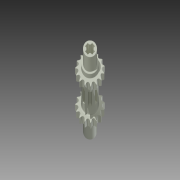
# Autodesk Inventor part: 1
Saved by Autodesk Inventor 2015 (Build 190159000, 159)
## iProperties
Created: 2016-01-25
Part Number: 1
Material: Plástico ABS
Document SubType Name: Modeling
Designer: Javier Pérez de Frutos
Density: 1.06 g/cm^3
Appearance: Suave - Marfil
z: 15,000 su
deje: 1,600 mm
rcanal: 0,500 mm
Dint: 13,500 mm
r3: 12,475 mm
Dcanal: 10,000 mm
Lcanal: 10,000 mm
L: 15,000 mm
Dext: 16,842 mm
Dr: 1,500 mm
Dp: 15,000 mm
r1: 1,124 mm
r2: 3,960 mm
chi: 124,00 gr
tau: 24,00 gr
p: 3,119 mm
Author: Javier Pérez de Frutos
Title: Piñón Tractor
Autodesk Inventor part; units mm, degrees
ref_plane "YZ Plane" through (0, 0, 0) normal (1, 0, 0) x (0, 1, 0)
ref_plane "XZ Plane" through (0, 0, 0) normal (0, 1, 0) x (-1, 0, 0)
ref_plane "XY Plane" through (0, 0, 0) normal (0, 0, 1) x (1, 0, 0)
sketch "Base" plane through (0, 0, 0) normal (0, 0, 1) x (1, 0, 0)
  circle A0 centre (0, 0) radius 7.5
  dimension "d0" = 15
  constraints: 1 centre point, 1 coincident
  measures "d0" diameter of A0
sketch "Tooth_drawing" plane through (0, 0, 0) normal (0, 0, 1) x (1, 0, 0)
  line L0 (0, 9) -> (0, -9)
  line L1 (-9, 0) -> (9, 0)
  line L2 (0, 0) -> (-1.7508, 8.2371)
  line L3 (0, 0) -> (1.7508, 8.2371)
  circle A0 centre (0, 7.5) radius 0.75
  arc A1 (-0.9925, 7.3464) -> (0.9925, 7.3464) centre (0, 7.8741) ccw
  line L4 (0, 7.8741) -> (-0.9925, 7.3464)
  line L5 (0, 7.8741) -> (0.9925, 7.3464)
  circle A2 centre (0, 0) radius 8.4211
  arc A3 (-0.9925, 7.3464) -> (-1.6459, 8.2587) centre (-4.7327, 5.3577) ccw
  arc A4 (1.6459, 8.2587) -> (0.9925, 7.3464) centre (4.7327, 5.3577) ccw
  dimension "d17" = 12
  dimension "d18" = 12
  dimension "d19" = 7.5
  dimension "d20" = 1.5
  dimension "d21" = 2.2482
  dimension "d22" = 62
  dimension "d23" = 62
  dimension "d25" = 16.8422
  constraints: 12 end point, 10 point on circle, 5 centre point, 3 point on line, 2 coincident, 2 midpoint, 2 tangent, 1 perpendicular, 1 vertical
  measures "d17" angle of L2 L0
  measures "d18" angle of L0 L3
  measures "d19" distance of point (0, 0) A0.centre
  measures "d20" diameter of A0
  measures "d21" diameter of A1
  measures "d22" angle of L0 L4
  measures "d23" angle of L0 L5
  measures "d25" diameter of A2
extrude "Tooth" add sketch "Tooth_drawing" along normal mid plane 15 contours A2 L3 L0 A1 A4 | A3 A1 L0 L2 A2
pattern_circular "Teeth" count 15 over 360 about axis through (0, 0, -10) along (0, 0, 1) of "Tooth"
sketch "Canal_drawing" plane through (0, 0, 0) normal (0, 1, 0) x (-1, 0, 0)
  line L0 (7.7013, 0) -> (-7.7013, 0)
  line L1 (-5.5, 5) -> (-6.75, 5)
  line L2 (-5, 4.5) -> (-5, 0)
  arc A0 (-8.4211, 5.228) -> (-6.75, 5) centre (-6.75, 11.2374) ccw
  line L3 (0, 7.5) -> (-6.75, 7.5)
  line L4 (0, 0) -> (0, 7.5)
  arc A1 (-6.75, 7.5) -> (-8.4211, 7.1913) centre (-6.75, 2.822) ccw
  line L5 (1.3412, 6.25) -> (-12.5756, 6.25)
  line L6 (-8.4211, 7.1913) -> (-8.4211, 5.228)
  line L7 (-5.5, -5) -> (-6.75, -5)
  line L8 (-5, -4.5) -> (-5, 0)
  arc A2 (-6.75, -5) -> (-8.4211, -5.228) centre (-6.75, -11.2374) ccw
  line L9 (0, -7.5) -> (-6.75, -7.5)
  line L10 (0, 0) -> (0, -7.5)
  arc A3 (-8.4211, -7.1913) -> (-6.75, -7.5) centre (-6.75, -2.822) ccw
  line L11 (-8.4211, -7.1913) -> (-8.4211, -5.228)
  line L12 (0, -15.7323) -> (0, 15.7323) projected
  arc A4 (-5.5, -5) -> (-5, -4.5) centre (-5.5, -4.5) ccw
  arc A5 (-5, 4.5) -> (-5.5, 5) centre (-5.5, 4.5) ccw
  point P0 (0, 0)
  point P1 (-5, 5)
  point P2 (-5, -5)
  dimension "d48" = 5
  dimension "d50" = 12.4747
  dimension "d53" = 6.75
  dimension "d54" = 6.75
  dimension "d56" = 6.75
  dimension "d57" = 4.678
  dimension "d58" = 12.5
  dimension "d59" = 8.4211
  dimension "d60" = 5
  dimension "d61" = 15
  dimension "d63" = 0.5
  constraints: 24 end point, 12 point on circle, 8 symmetric about line, 6 centre point, 6 tangent, 5 point on line, 4 horizontal, 2 midpoint, 1 coincident, 1 equal radius, 1 perpendicular, 1 vertical, 2 other
  measures "d48" distance from line of point (0, 0) L2
  measures "d50" diameter of A0
  measures "d53" distance from line of L4 A0.centre
  measures "d54" distance from line of L1.end L4
  measures "d56" horizontal distance of point (0, 0) A1.centre
  measures "d57" radius of A1
  measures "d58" diameter of L5.start L0
  measures "d59" distance from line of L6.start L4
  measures "d60" distance of point (-5, 5) L2.end
  measures "d61" diameter of L3 L0
  measures "d63" radius of A4
revolve "Canal" cut sketch "Canal_drawing" angle 360 about axis through (0, 0, -10) along (0, 0, 1) keep common part
sketch "Axis_drawing" plane through (0, 0, 0) normal (0, 0, 1) x (1, 0, 0)
  arc A0 (-1.6, -1.2) -> (-1.6, 1.2) centre (0, 0) ccw
  line L0 (-1.6, 1.2) -> (-1.6, -1.2)
  dimension "d64" = 4
  dimension "d65" = 1.6
  constraints: 2 end point, 2 point on circle, 1 centre point, 1 coincident, 1 vertical
  measures "d64" diameter of A0
  measures "d65" distance from line of point (0, 0) L0
extrude "Axis" [suppressed]
sketch "Holes_drawing" plane through (0, 0, 0) normal (0, 0, 1) x (1, 0, 0)
  circle A0 centre (0, 0) radius 5 projected
  circle A1 centre (0, 0) radius 5 projected
  arc A2 (-1.6, -1.2) -> (-1.6, 1.2) centre (0, 0) ccw projected
  line L0 (1.9182, -4.6174) -> (0.7673, -1.847)
  circle A3 centre (0, 0) radius 3.5
  circle A4 centre (-3.5, 0) radius 0.75
  circle A5 centre (-1.75, -3.0311) radius 0.75
  circle A6 centre (1.75, -3.0311) radius 0.75
  circle A7 centre (3.5, 0) radius 0.75
  circle A8 centre (1.75, 3.0311) radius 0.75
  circle A9 centre (-1.75, 3.0311) radius 0.75
  dimension "d68" = 1.5
  dimension "d71" = 360
  constraints: 6 centre point, 2 end point, 1 coincident, 1 horizontal alignment, 1 point on circle, 19 other
  measures "d68" diameter of A4
extrude "Holes" [suppressed]
sketch "Boceto9" plane through (0, 0, 0) normal (0, 0, 1) x (1, 0, 0)
  circle A0 centre (0, 0) radius 4
  dimension "d81" = 8
  constraints: 1 centre point, 1 coincident
  measures "d81" diameter of A0
sketch "Boceto10" plane through (0, 0, 0) normal (0, 0, 1) x (1, 0, 0)
  circle A0 centre (0, 0) radius 5
  dimension "d84" = 10
  constraints: 1 centre point, 1 coincident
  measures "d84" diameter of A0
extrude "Extrusión10" add sketch "Boceto10" along normal mid plane 18
extrude "Extrusión9" add sketch "Boceto9" along normal mid plane 28
sketch "Boceto8" plane through (0, 0, 0) normal (1, 0, 0) x (0, 1, 0)
  line L0 (-6.7222, 2.8333) -> (-3.5, 2.8333)
  line L1 (-3.5, 2.8333) -> (-3.5, -2.1667)
  line L2 (-3.5, -2.1667) -> (-6.7222, -2.1667)
  line L3 (-6.7222, -2.1667) -> (-6.7222, 2.8333)
  line L4 (0, 13.3538) -> (0, -28.5984)
  point P0 (0, 0)
  dimension "d75" = 5
  dimension "d76" = 7
  constraints: 10 end point, 2 parallel, 2 vertical, 1 horizontal, 1 perpendicular
  measures "d75" distance of L2.end L0.start
  measures "d76" diameter of L1 L4
revolve "EncoderPulse" cut sketch "Boceto8" angle 22.5 mid plane about axis through (0, 0, 13.3538) along (0, 0, -1)
pattern_circular "Encoder" count 8 over 360 about axis through (0, 0, -10) along (0, 0, 1) of "EncoderPulse"
sketch "Boceto11" plane through (0, 0, 14) normal (0, 0, 1) x (1, 0, 0)
  circle A0 centre (0, 0) radius 5
  circle A1 centre (0, 0) radius 4
  circle A2 centre (0, 0) radius 5
  line L0 (1, -2.75) -> (-1, -2.75)
  line L1 (-1, 2.75) -> (1, 2.75)
  line L2 (0, -5.7465) -> (0, 6.3823)
  line L3 (9.3922, 0) -> (-10.1811, 0)
  line L4 (-2.75, -1) -> (-2.75, 1)
  line L5 (2.75, 1) -> (2.75, -1)
  line L6 (2.75, -1) -> (1, -1)
  line L7 (-1, -1) -> (-2.75, -1)
  line L8 (-1, -2.75) -> (-1, -1)
  line L9 (-1, 1) -> (-1, 2.75)
  line L10 (-2.75, 1) -> (-1, 1)
  line L11 (1, 1) -> (2.75, 1)
  line L12 (1, 2.75) -> (1, 1)
  line L13 (1, -1) -> (1, -2.75)
  line L14 (-1.1, -1.1) -> (-2.85, -1.1)
  line L15 (-2.85, -1.1) -> (-2.85, 1.1)
  line L16 (-2.85, 1.1) -> (-1.1, 1.1)
  line L17 (-1.1, 1.1) -> (-1.1, 2.85)
  line L18 (-1.1, 2.85) -> (1.1, 2.85)
  line L19 (1.1, 2.85) -> (1.1, 1.1)
  line L20 (1.1, 1.1) -> (2.85, 1.1)
  line L21 (2.85, 1.1) -> (2.85, -1.1)
  line L22 (2.85, -1.1) -> (1.1, -1.1)
  line L23 (1.1, -1.1) -> (1.1, -2.85)
  line L24 (1.1, -2.85) -> (-1.1, -2.85)
  line L25 (-1.1, -2.85) -> (-1.1, -1.1)
  circle A3 centre (0, 0) radius 2
  circle A4 centre (0, 0) radius 2.1
  dimension "d94" = 2
  dimension "d95" = 2
  dimension "d96" = 5.5
  dimension "d97" = 5.5
  dimension "d98" = 0.1
  dimension "d99" = 4
  dimension "d100" = 0.1
  constraints: 52 end point, 20 parallel, 8 perpendicular, 5 centre point, 5 horizontal, 2 coincident, 2 vertical, 11 other
  measures "d94" distance of L1.start L1.end
  measures "d95" distance of L4.start L4.end
  measures "d96" distance between parallel lines of L1 L0
  measures "d97" distance between parallel lines of L4 L5
  measures "d98" distance between parallel lines of L8 L25
  measures "d99" diameter of A3
  measures "d100" radial gap between concentric circles of A3 A4
extrude "Extrusión11" cut sketch "Boceto11" against normal blind 12 contours L21 L22 A4 L6 L5 L3 | L3 L5 L11 A4 L20 L21 | L18 L19 A4 L12 L1 L2 | L2 L1 L9 A4 L17 L18 | L24 L25 A4 L8 L0 L2 | L2 L0 L13 A4 L23 L24 | L5 L6 A4 L3 | L3 A4 L11 L5 | L15 L16 A4 L10 L4 L3 | L3 L4 L7 A4 L14 L15 | L2 A4 L9 L1 | L1 L12 A4 L2 | L2 A4 L13 L0 | L0 L8 A4 L2 | A4 L6 A3 L3 | L3 A3 L11 A4 | A4 L11 A3 L20 | L20 A3 L19 A4 | A4 L23 A3 L22 | L22 A3 L6 A4 | L4 L10 A4 L3 | L3 A4 L7 L4 | A4 L12 A3 L2 | L2 A3 L9 A4 | A4 L9 A3 L17 | L17 A3 L16 A4 | L19 A3 L12 A4 | A4 L8 A3 L2 | L2 A3 L13 A4 | A4 L13 A3 L23 | A4 L14 A3 L25 | L25 A3 L8 A4 | A3 L6 L13 L2 L3 | L3 L2 A3 L12 L11 | A3 L11 L12 L19 L20 | L20 L19 A3 | A3 L23 L22 | L22 L23 A3 L13 L6 | A4 L10 A3 L3 | L3 A3 L7 A4 | A4 L7 A3 L14 | L16 A3 L10 A4 | L2 L3 A3 L10 L9 | A3 L9 L10 L16 L17 | L17 L16 A3 | A3 L8 L7 L3 L2 | A3 L14 L25 | L25 L14 A3 L7 L8
equation "\"d0\" = Dp"
equation "\"d17\" = 0.5 * tau"
equation "\"d18\" = 0.5 * tau"
equation "\"d19\" = 0.5 * Dp"
equation "\"d20\" = Dr"
equation "\"d21\" = 2 * r1"
equation "\"d22\" = 0.5 * chi"
equation "\"d23\" = 0.5 * chi"
equation "\"d25\" = Dext"
equation "\"d35\" = L"
equation "\"d48\" = 0.5 * Dcanal"
equation "\"d50\" = r3"
equation "\"d53\" = 0.5 * Dint"
equation "\"d56\" = 0.5 * Dint"
equation "\"d58\" = 0.5 * L + 0.5 * Lcanal"
equation "\"d59\" = 0.5 * Dext"
equation "\"d60\" = 0.5 * Lcanal"
equation "\"d61\" = L"
equation "\"d63\" = rcanal"
equation "\"d64\" = Deje"
equation "\"d65\" = deje"
equation "\"d77\" = pulsesAngle"
equation "\"Dr\" = 1.5"
equation "\"Dp\" = 15"
equation "\"d24\" = 2 * r2"
equation "\"d26\" = 2 * r2"
equation "\"L\" = 15"
equation "\"Lcanal\" = 10"
equation "\"Dcanal\" = 10"
equation "\"r3\" = 4 * p"
equation "\"Dint\" = Dp - Dr"
equation "\"d55\" = r3"
equation "\"rcanal\" = 0.5"
equation "\"Deje\" = 4"
equation "\"deje\" = 1.6"
equation "\"tau\" = 24deg"
equation "\"r1\" = 1.124117"
equation "\"chi\" = 124deg"
equation "\"Dext\" = 16.84218"
equation "\"pulsesAngle\" = 22.5deg"
equation "\"r2\" = 3.96"
equation "\"p\" = 3.118675"
